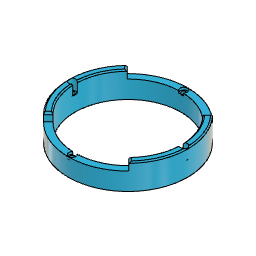
Structure_hublot_KOSMOS3-0 (Autodesk Fusion 360 design; units mm, degrees)
Autodesk Fusion 360 part; units mm, degrees
sketch "Esquisse1" plane through (0, 0, 0) normal (0, 0, 1) x (1, 0, 0)
  circle A0 centre (0, 0) radius 50.6
  circle A1 centre (0, 0) radius 44.95
  dimension "d1" = 101.2
  dimension "d123" = 89.9
  constraint coincident A0.centre A1.centre
  measures "d1" diameter of A0
  measures "d123" diameter of A1
extrude "Extrusion2" add sketch "Esquisse1" along normal blind 15
sketch "Esquisse10" plane through (0, 0, 15) normal (0, 0, 1) x (-1, 0, 0)
  circle A0 centre (0, -47.3) radius 1.9
  line L0 (0, -50.6) -> (-13, -50.6) construction
  circle A1 centre (47.3, 0) radius 1.9
  circle A2 centre (0, 47.3) radius 1.9
  circle A3 centre (-47.3, 0) radius 1.9
  circle A4 centre (0, 0) radius 50.6
  circle A5 centre (0, 0) radius 44.95
  dimension "d116" = 3.8
  dimension "d118" = 3.3
  dimension "d120" = 360
  constraint coincident L0.start A4
  constraint tangent L0 A4
  constraint horizontal L0
  measures "d116" diameter of A0
  measures "d118" distance of A0.centre L0
extrude "Extrusion12" cut sketch "Esquisse10" against normal blind 35 contours A0 | A1 | A2 | A3
sketch "Esquisse12" plane through (0, 0, 15) normal (0, 0, 1) x (-1, 0, 0)
  circle A0 centre (-47.3, 0) radius 1.9
  circle A1 centre (0, 47.3) radius 1.9
  circle A2 centre (0, -47.3) radius 1.9
  circle A3 centre (47.3, 0) radius 1.9
  circle A4 centre (0, 0) radius 44.95
  circle A5 centre (0, 0) radius 50.6
  line L0 (0, 0) -> (45.3212, -45.3212) construction
  line L1 (0, 0) -> (64.0938, 0) construction
  line L2 (40.2866, -39.5795) -> (25.4205, -24.7134) construction
  line L3 (36.1314, -35.4243) -> (32.136, -31.4289)
  line L4 (36.1314, 35.4243) -> (32.136, 31.4289)
  line L5 (-36.1314, 35.4243) -> (-32.136, 31.4289)
  line L6 (-36.1314, -35.4243) -> (-32.136, -31.4289)
  line L7 (0, 0) -> (-50.6611, -50.6611) construction
  line L8 (0, 0) -> (71.6455, 0) construction
  line L9 (0, 0) -> (-40.5771, 40.5771) construction
  line L10 (0, 0) -> (57.3847, 0) construction
  line L11 (0, 0) -> (45.4395, 45.4395) construction
  line L12 (0, 0) -> (64.2612, 0) construction
  circle A6 centre (0, 0) radius 50.6
  circle A7 centre (0, 0) radius 44.95
  dimension "d124" = 45
  dimension "d125" = 0.5
  dimension "d143" = 135
  dimension "d144" = 0.5
  dimension "d145" = 135
  dimension "d146" = 0.5
  dimension "d147" = 45
  dimension "d148" = 0.5
  constraint horizontal L1
  constraint coincident A4.centre A5.centre
  constraint parallel L0 L2
  constraint coincident A5 L3.start
  constraint coincident L2 L3.start
  constraint coincident L2 L3.end
  constraint coincident A4 L3.end
  constraint horizontal L8
  constraint horizontal L10
  constraint horizontal L12
  constraint concentric A4 A7
  constraint coincident L4.start A6
  constraint coincident L4.end A7
  constraint coincident L3.end A7
  constraint coincident L3.start A6
  constraint coincident L6.start A6
  constraint coincident L6.end A7
  constraint coincident L5.start A6
  constraint coincident L5.end A7
  measures "d124" angle of L0 L1
  measures "d125" distance of L0 L2
  measures "d143" angle of L7 L8
  measures "d144" distance of L6 L7
  measures "d145" angle of L9 L10
  measures "d146" distance of L5 L9
  measures "d147" angle of L11 L12
  measures "d148" distance of L4 L11
extrude "Extrusion16" add sketch "Esquisse12" along normal blind 6.7 contours A4 A5 L3 L4 A6 A7 | A4 A5 L5 L6 A6 A7
sketch "Esquisse13" plane through (0, 0, 15) normal (0, 0, 1) x (-1, 0, 0)
  arc A0 (-32.136, -31.4289) -> (32.136, -31.4289) centre (0, 0) ccw
  arc A1 (-36.1314, -35.4243) -> (36.1314, -35.4243) centre (0, 0) ccw
  circle A2 centre (0, -47.3) radius 1.9
  circle A3 centre (0, -47.3) radius 3
  circle A4 centre (0, 47.3) radius 3
  line L0 (-32.136, -31.4289) -> (-36.1314, -35.4243)
  line L1 (36.1314, -35.4243) -> (32.136, -31.4289)
  dimension "d131" = 6
  dimension "d133" = 360
  constraint concentric A2 A3
  measures "d131" diameter of A3
extrude "Extrusion14" cut sketch "Esquisse13" against normal blind 2 contours A0 A3 | A4 picked at (1.1245, -45.1712)
sketch "Esquisse14" plane through (0, 0, 21.7) normal (0, 0, 1) x (-1, 0, 0)
  circle A0 centre (-47.3, 0) radius 3
  circle A1 centre (47.3, 0) radius 3
  circle A2 centre (0, 0) radius 44.95
  circle A3 centre (0, 0) radius 50.6
  circle A4 centre (47.3, 0) radius 1.9
  circle A5 centre (47.3, 0) radius 1.9
  arc A6 (36.1314, -35.4243) -> (36.1314, 35.4243) centre (0, 0) ccw
  line L0 (36.1314, 35.4243) -> (32.136, 31.4289)
  arc A7 (32.136, -31.4289) -> (32.136, 31.4289) centre (0, 0) ccw
  line L1 (32.136, -31.4289) -> (36.1314, -35.4243)
  dimension "d136" = 6
  dimension "d138" = 360
  measures "d136" diameter of A0
extrude "Extrusion15" cut sketch "Esquisse14" against normal blind 9 contours A0 A2 | A1 A2 A7 | A1 A2 A7 | A4 A5 picked at (-46.7306, 0)
chamfer "Chanfrein6" distance 1.5 angle 45 4 edges at (-34.1337, -33.4266, 21.7) (-34.1337, 33.4266, 21.7) (34.1337, 33.4266, 21.7) (34.1337, -33.4266, 21.7)
chamfer "Chanfrein7" distance 1 angle 45 6 edges at (41.5632, 17.1172, 21.7) (-41.5632, -17.1172, 21.7) (-41.5632, 17.1172, 21.7) (-50.6, 0, 21.7) (50.6, 0, 21.7) (41.5632, -17.1172, 21.7)
